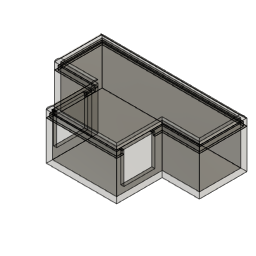
door sensor (Autodesk Fusion 360 design; units mm, degrees)
Autodesk Fusion 360 part; units mm, degrees
sketch "Sketch1" plane through (0, 0, 0) normal (0, 0, 1) x (1, 0, 0)
  line L0 (0, 0) -> (70, 0)
  line L1 (70, 0) -> (70, 45)
  line L2 (70, 45) -> (0, 45)
  line L3 (0, 45) -> (0, 0)
  line L4 (0, 45) -> (0, 22) construction
  line L5 (35, 45) -> (35, 0) construction
  line L6 (35, 0) -> (52, 0) construction
  line L7 (35, 0) -> (18, 0) construction
  line L8 (0, 22) -> (18, 22)
  line L9 (18, 22) -> (18, 0)
  line L10 (52, 0) -> (52, 22)
  line L11 (52, 22) -> (70, 22)
  dimension "d1" = 70
  dimension "d2" = 45
  dimension "d3" = 23
  dimension "d4" = 17
  dimension "d5" = 17
  constraint horizontal L0
  constraint vertical L1
  constraint horizontal L2
  constraint vertical L3
  constraint coincident L0.start L3.end
  constraint perpendicular L2 L4
  constraint midpoint L2 L5.start
  constraint midpoint L0 L5.end
  constraint perpendicular L5 L6
  constraint perpendicular L5 L7
  constraint perpendicular L3 L8
  constraint perpendicular L7 L9
  constraint perpendicular L8 L10
  constraint perpendicular L10 L11
  measures "d1" distance of L0.start L0.end
  measures "d2" distance of L0.start L2.end
  measures "d3" distance of L2.end L4.end
  measures "d4" distance of L5.end L6.end
  measures "d5" distance of L5.end L7.end
extrude "Extrude1" add sketch "Sketch1" along normal blind 24 contours L0 L1 L2 L3 L8 L9 L10 L11 makes body 1
shell "Shell1" thickness 1.5 removed faces 0 bodies 1
ref_plane "WorkPlane1" through (52, 11, 12) normal (1, 0, 0) x (0, 1, 0)
sketch "Sketch2" plane through (52, 11, 12) normal (1, 0, 0) x (0, 1, 0)
  line L0 (12.5, -10.5) -> (32.5, -10.5)
  line L1 (32.5, -10.5) -> (12.5, -10.5)
  line L2 (12.5, -10.5) -> (-9.5, -10.5)
  line L3 (-9.5, -10.5) -> (12.5, -10.5)
  line L4 (-9.5, -10.5) -> (-9.5, -6.5)
  line L5 (-9.5, -10.5) -> (-8.5, -10.5)
  line L6 (-9.5, -10.5) -> (6.5, -10.5)
  line L7 (-9.5, -6.5) -> (-9.5, 9)
  line L8 (-8.5, -6.5) -> (6.5, -6.5)
  line L9 (6.5, -6.5) -> (6.5, 9)
  line L10 (6.5, 9) -> (-8.5, 9)
  line L11 (-8.5, 9) -> (-8.5, -6.5)
  dimension "d10" = 4
  dimension "d11" = 1
  dimension "d12" = 16
  dimension "d13" = 15.5
  constraint coincident L2.end L3.start
  constraint perpendicular L3 L4
  constraint perpendicular L4 L5
  constraint perpendicular L4 L6
  constraint perpendicular L6 L7
  constraint horizontal L8
  constraint vertical L9
  constraint horizontal L10
  constraint vertical L11
  measures "d10" distance of L2.end L4.end
  measures "d11" distance of L2.end L5.end
  measures "d12" distance of L2.end L6.end
  measures "d13" distance of L4.end L7.end
extrude "Extrude2" cut sketch "Sketch2" against normal blind 43 bodies 1
fillet "Fillet1" radius 0.01 4 edges at (51.25, 17.5, 21) (18.75, 17.5, 21) (51.25, 2.5, 21) (18.75, 2.5, 21) on bodies 1
extrude "Extrude3" cut 1 faces at (46.6667, 45, 16) along direction (0, -1, 0) blind 0.5 on bodies 1 bodies 1
ref_plane "WorkPlane2" through (35, 22.25, 19) normal (0, 0, 1) x (1, 0, 0)
split "Split1" by plane through (35, 22.25, 19) normal (0, 0, 1) bodies 1 makes body 2 at (29.3333, 37, 24)
sketch "Sketch3" plane through (35, 22.25, 19) normal (0, 0, 1) x (1, 0, 0)
  line L0 (15.5, -4.75) -> (17, -4.75)
  line L1 (17, -4.75) -> (17, -0.25)
  line L2 (17, -0.25) -> (35, -0.25)
  line L3 (35, -0.25) -> (35, 22.25)
  line L4 (35, 22.25) -> (-35, 22.25)
  line L5 (-35, 22.25) -> (-35, -0.25)
  line L6 (-35, -0.25) -> (-17, -0.25)
  line L7 (-17, -0.25) -> (-17, -4.75)
  line L8 (-17, -4.75) -> (-15.5, -4.75)
  line L9 (-15.5, -4.75) -> (-15.5, 1.25)
  line L10 (-15.5, 1.25) -> (-33.5, 1.25)
  line L11 (-33.5, 1.25) -> (-33.5, 21.25)
  line L12 (-33.5, 21.25) -> (33.5, 21.25)
  line L13 (33.5, 21.25) -> (33.5, 1.25)
  line L14 (33.5, 1.25) -> (15.5, 1.25)
  line L15 (15.5, 1.25) -> (15.5, -4.75)
  line L16 (17, -19.75) -> (15.5, -19.75)
  line L17 (15.5, -19.75) -> (15.5, -20.75)
  line L18 (15.5, -20.75) -> (-15.5, -20.75)
  line L19 (-15.5, -20.75) -> (-15.5, -19.75)
  line L20 (-15.5, -19.75) -> (-17, -19.75)
  line L21 (-17, -19.75) -> (-17, -22.25)
  line L22 (-17, -22.25) -> (17, -22.25)
  line L23 (17, -22.25) -> (17, -19.75)
  line L24 (-16.15, -4.75) -> (-16.15, 0.6)
  line L25 (-16.15, 0.6) -> (-34.15, 0.6)
  line L26 (-34.15, 0.6) -> (-34.15, 21.9)
  line L27 (-34.15, 21.9) -> (34.15, 21.9)
  line L28 (34.15, 21.9) -> (34.15, 0.6)
  line L29 (34.15, 0.6) -> (16.15, 0.6)
  line L30 (16.15, 0.6) -> (16.15, -4.75)
  line L31 (16.15, -19.75) -> (16.15, -21.4)
  line L32 (16.15, -21.4) -> (-16.15, -21.4)
  line L33 (-16.15, -21.4) -> (-16.15, -19.75)
  dimension "d21" = -0.65
  dimension "d22" = -0.65
extrude "Extrude4" add sketch "Sketch3" along normal blind 2 contours L0 L8 L9 L10 L11 L12 L13 L14 L15 L24 L25 L26 L27 L28 L29 L30 | L16 L17 L18 L19 L20 L31 L32 L33 bodies 1
combine "Combine1" operation cut target body 2 tool bodies 1 keep tools
fillet "Fillet2" radius 1.5 8 edges at (35, 44.5, 24) (0, 33.25, 24) (9, 22, 24) (18, 11, 24) (35, 0, 24) (52, 11, 24) (61, 22, 24) (70, 33.25, 24) on bodies 2
extrude "Extrude5" add 1 faces at (46.6667, 44.5, 6.3333) along direction (0, 1, 0) blind 0.5 on bodies 1 bodies 1
extrude "Extrude6" add 1 faces at (46.6667, 44.5, 20.1667) along direction (0, 1, 0) blind 0.5 on bodies 2 bodies 2
extrude "Extrude7" cut 1 faces at (51.2167, 17.5, 10) along direction (0, 1, 0) blind 1 on bodies 1 bodies 1
extrude "Extrude8" cut 1 faces at (18.7833, 17.5, 10) along direction (0, 1, 0) blind 1 on bodies 1 bodies 1
extrude "Extrude9" cut 2 faces at (51.7167, 17.5, 19.6633) (18.5667, 17.5, 19.6633) along direction (0, 1, 0) blind 1 on bodies 2 bodies 2
extrude "Extrude10" add 2 faces at (51.7167, 2.5, 20.3267) (18.5667, 2.5, 20.3267) along direction (0, 1, 0) blind 1 on bodies 2 bodies 2
extrude "Extrude11" add 2 faces at (18.7833, 2.5, 10) (51.2167, 2.5, 10) along direction (0, 1, 0) blind 1 on bodies 1 bodies 1
named bodies: "bot", "top"
